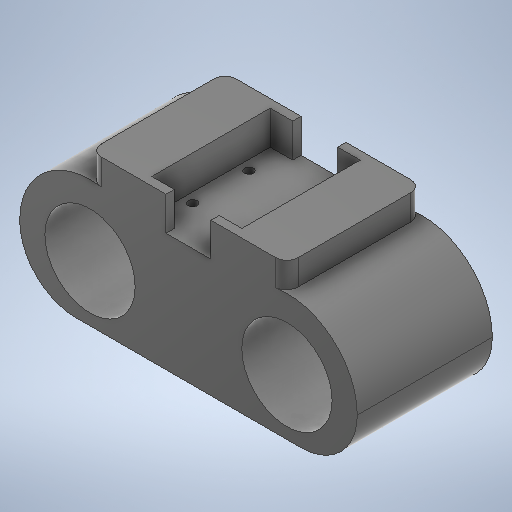
# Autodesk Inventor part: Space Craft Braket
Saved by Autodesk Inventor 2026.2 (Build 302298010, 298A)
## iProperties
Created: 2026-04-29
Part Number: Space Craft Braket
Material: ABS Plastic
Document SubType Name: Modeling
Designer: chanh
Density: 1.06 g/cm^3
Appearance: Smooth - White
Author: chanh
Autodesk Inventor part; units mm, degrees
ref_plane "YZ Plane" through (0, 0, 0) normal (1, 0, 0) x (0, 1, 0)
ref_plane "XZ Plane" through (0, 0, 0) normal (0, 1, 0) x (-1, 0, 0)
ref_plane "XY Plane" through (0, 0, 0) normal (0, 0, 1) x (1, 0, 0)
sketch "Sketch1" plane through (0, 0, 0) normal (0, 0, 1) x (1, 0, 0)
  line L0 (-35, 0) -> (35, 0) construction
  circle A0 centre (-35, 0) radius 16.05
  circle A1 centre (35, 0) radius 16.05
  arc A2 (-20, -20) -> (-50, -20) centre (-35, 0) ccw
  arc A3 (50, -20) -> (20, -20) centre (35, 0) ccw
  line L1 (-35, 25) -> (35, 25)
  line L2 (-50, -20) -> (50, -20)
  point P0 (0, 0)
  point P1 (0, 0)
  dimension "d0" = 70
  dimension "d1" = 32.1
  dimension "d3" = 50
  dimension "d38" = 20
  constraints: 6 end point, 6 point on circle, 5 coincident, 4 centre point, 3 horizontal, 2 equal radius, 2 point on line, 1 midpoint, 1 tangent
  measures "d0" distance of L0.start L0.end
  measures "d1" diameter of A0
  measures "d3" diameter of A2
  measures "d38" distance between parallel lines of L0 L2
extrude "Extrusion1" add sketch "Sketch1" along normal mid plane 48
fillet "Fillet3" radius 20 2 edges at (50, -20, 0) (-50, -20, 0)
sketch "Sketch10" plane through (-35, 25, 24) normal (0, 1, 0) x (1, 0, 0)
  line L0 (0, 48) -> (0, 0) projected
  line L1 (70, 0) -> (0, 0) projected
  line L2 (70, 48) -> (70, 0) projected
  line L3 (0, 48) -> (70, 48) projected
  point P0 (35, 24)
extrude "Extrusion4" add sketch "Sketch10" along normal blind 9
sketch "Sketch11" plane through (-35, 34, 24) normal (0, 1, 0) x (1, 0, 0)
  line L0 (19, 2.95) -> (51, 2.95)
  line L1 (51, 2.95) -> (51, 45.05)
  line L2 (51, 45.05) -> (19, 45.05)
  line L3 (19, 45.05) -> (19, 2.95)
  line L4 (19, 2.95) -> (51, 45.05) construction
  line L5 (51, 2.95) -> (19, 45.05) construction
  line L6 (0, 48) -> (0, 0) projected
  line L7 (0, 0) -> (70, 0) projected
  line L8 (70, 0) -> (70, 48) projected
  line L9 (70, 48) -> (0, 48) projected
  line L10 (27, 48) -> (43, 48)
  line L11 (43, 48) -> (43, 45.05)
  line L12 (43, 45.05) -> (27, 45.05)
  line L13 (27, 45.05) -> (27, 48)
  line L14 (27, 2.95) -> (27, 0)
  line L15 (35, 24) -> (35, 47.5578) construction
  line L16 (43, 2.95) -> (43, 0)
  point P0 (35, 45.05)
  point P1 (43, 0)
  point P2 (43, 2.95)
  dimension "d49" = 32
  dimension "d50" = 42.1
  dimension "d53" = 16
  constraints: 26 end point, 4 parallel, 4 point on line, 3 midpoint, 3 perpendicular, 2 horizontal, 2 symmetric about line, 1 collinear, 1 vertical, 1 vertical alignment
  measures "d49" distance of L1.end L2.end
  measures "d50" distance of L0.end L1.end
  measures "d53" distance between parallel lines of L11 L13
extrude "Extrusion5" cut sketch "Sketch11" against normal blind 12 contours L3 L2 L1 L0 | L0 L16 L7 L14 | L13 L9 L11 L2
sketch "Sketch12" plane through (-40, -20, -24) normal (0, -1, 0) x (1, 0, 0)
  line L0 (27.5, 14) -> (52.5, 14) construction
  line L1 (52.5, 14) -> (52.5, 34) construction
  line L2 (52.5, 34) -> (27.5, 34) construction
  line L3 (27.5, 34) -> (27.5, 14) construction
  line L4 (27.5, 14) -> (52.5, 34) construction
  line L5 (52.5, 14) -> (27.5, 34) construction
  point P0 (40, 24)
  dimension "d54" = 25
  dimension "d55" = 20
  constraints: 12 end point, 4 coincident, 2 midpoint, 2 parallel, 1 horizontal, 1 perpendicular
  measures "d54" distance of L0.start L0.end
  measures "d55" distance of L0.end L1.end
hole "Hole4" at (-12.5, -20, 10) at (12.5, -20, 10) at (12.5, -20, -10) at (-12.5, -20, -10) direction (0, 1, 0) diameter 3.2 end through all counterbore diameter 6.5 counterbore depth 20
fillet "Fillet4" radius 4 4 edges at (35, 29.5, 24) (35, 29.5, -24) (-35, 29.5, 24) (-35, 29.5, -24)
body "Solid1"
